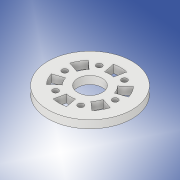
# Autodesk Inventor part: Flexspline
Saved by Autodesk Inventor 2017 SP1 (Build 210196100, 196)
## iProperties
Created: 2017-07-11
Part Number: Flexspline
Material: ABS Plastic
Document SubType Name: Modeling
Designer: zallen
Density: 1.06 g/cm^3
Appearance: CR White
Author: zallen
Autodesk Inventor part; units mm, degrees
ref_plane "YZ Plane" through (0, 0, 0) normal (1, 0, 0) x (0, 1, 0)
ref_plane "XZ Plane" through (0, 0, 0) normal (0, 1, 0) x (-1, 0, 0)
ref_plane "XY Plane" through (0, 0, 0) normal (0, 0, 1) x (1, 0, 0)
sketch "Sketch3" plane through (0, 0, 0) normal (0, 1, 0) x (-1, 0, 0)
  circle A0 centre (0, 0) radius 11
  circle A1 centre (0, 0) radius 17.5 construction
  circle A2 centre (0, 0) radius 27.5 construction
  circle A3 centre (0, 0) radius 37.5
  line L0 (-6, 26.8375) -> (-4, 17.0367)
  line L1 (6, 26.8375) -> (4, 17.0367)
  arc A4 (6, 26.8375) -> (-6, 26.8375) centre (0, 0) ccw
  arc A5 (4, 17.0367) -> (-4, 17.0367) centre (0, 0) ccw
  circle A6 centre (0, 0) radius 22.5 construction
  line L2 (5.0001, 21.9374) -> (16.4983, 15.2989) construction
  line L3 (10.7492, 18.6181) -> (11.25, 19.4856) construction
  circle A7 centre (11.25, 19.4856) radius 2.5
  circle A8 centre (-11.25, 19.4856) radius 2.5
  circle A9 centre (-22.5, 0) radius 2.5
  circle A10 centre (-11.25, -19.4856) radius 2.5
  circle A11 centre (11.25, -19.4856) radius 2.5
  circle A12 centre (22.5, 0) radius 2.5
  arc A13 (-20.2419, 18.6149) -> (-26.2419, 8.2226) centre (0, 0) ccw
  line L4 (-20.2419, 18.6149) -> (-12.7542, 11.9825)
  line L5 (-26.2419, 8.2226) -> (-16.7542, 5.0543)
  arc A14 (-12.7542, 11.9825) -> (-16.7542, 5.0543) centre (0, 0) ccw
  arc A15 (-26.2419, -8.2226) -> (-20.2419, -18.6149) centre (0, 0) ccw
  line L6 (-26.2419, -8.2226) -> (-16.7542, -5.0543)
  line L7 (-20.2419, -18.6149) -> (-12.7542, -11.9825)
  arc A16 (-16.7542, -5.0543) -> (-12.7542, -11.9825) centre (0, 0) ccw
  arc A17 (-6, -26.8375) -> (6, -26.8375) centre (0, 0) ccw
  line L8 (-6, -26.8375) -> (-4, -17.0367)
  line L9 (6, -26.8375) -> (4, -17.0367)
  arc A18 (-4, -17.0367) -> (4, -17.0367) centre (0, 0) ccw
  arc A19 (20.2419, -18.6149) -> (26.2419, -8.2226) centre (0, 0) ccw
  line L10 (20.2419, -18.6149) -> (12.7542, -11.9825)
  line L11 (26.2419, -8.2226) -> (16.7542, -5.0543)
  arc A20 (12.7542, -11.9825) -> (16.7542, -5.0543) centre (0, 0) ccw
  arc A21 (26.2419, 8.2226) -> (20.2419, 18.6149) centre (0, 0) ccw
  line L12 (26.2419, 8.2226) -> (16.7542, 5.0543)
  line L13 (20.2419, 18.6149) -> (12.7542, 11.9825)
  arc A22 (16.7542, 5.0543) -> (12.7542, 11.9825) centre (0, 0) ccw
  point P0 (-16.4983, 15.2989)
  point P1 (-21.4984, -6.6385)
  point P2 (-5.0001, -21.9374)
  point P3 (16.4983, -15.2989)
  point P4 (21.4984, 6.6385)
  dimension "d16" = 22
  dimension "d17" = 35
  dimension "d18" = 55
  dimension "d19" = 75
  dimension "d20" = 6
  dimension "d21" = 4
  dimension "d22" = 6
  dimension "d23" = 4
  dimension "d28" = 45
  dimension "d29" = 5
  dimension "d32" = 360
  dimension "d38" = 360
  constraints: 31 point on circle, 28 end point, 23 centre point, 7 point on line, 6 coincident, 3 concentric, 1 midpoint, 1 perpendicular, 80 other
  measures "d16" diameter of A0
  measures "d17" diameter of A1
  measures "d18" diameter of A2
  measures "d19" diameter of A3
  measures "d20" horizontal distance of point (0, 0) L0.start
  measures "d21" horizontal distance of point (0, 0) L0.end
  measures "d22" horizontal distance of point (0, 0) L1.start
  measures "d23" horizontal distance of point (0, 0) L1.end
  measures "d28" diameter of A6
  measures "d29" diameter of A7
extrude "Extrusion4" add sketch "Sketch3" along normal blind 7
body "Solid1"
